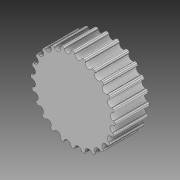
# Autodesk Inventor part: Timing Pulley Generator
Saved by Autodesk Inventor 2022 (Build 260153000, 153)
## iProperties
Created: 2022-01-03
Part Number: Timing Pulley Generator
Material: Generic
Document SubType Name: Modeling
Density: 1 g/cm^3
Appearance: Default
Autodesk Inventor part; units mm, degrees
ref_plane "YZ Plane" through (0, 0, 0) normal (1, 0, 0) x (0, 1, 0)
ref_plane "XZ Plane" through (0, 0, 0) normal (0, 1, 0) x (-1, 0, 0)
ref_plane "XY Plane" through (0, 0, 0) normal (0, 0, 1) x (1, 0, 0)
sketch "Sketch1" plane through (0, 0, 0) normal (0, 0, 1) x (1, 0, 0)
  circle A0 centre (0, 0) radius 11.4592
  dimension "d0" = 22.9183
  constraints: 1 centre point, 1 coincident
  measures "d0" diameter of A0
extrude "Base" add sketch "Sketch1" along normal mid plane 9
sketch "Sketch2" plane through (0, 0, 4.5) normal (0, 0, 1) x (1, 0, 0)
  arc A0 (0.3421, 10.8788) -> (0, 10.8842) centre (0, 0) ccw
  arc A1 (0.7166, 10.2636) -> (0.3421, 10.8788) centre (0.3286, 10.449) ccw
  arc A2 (0.7166, 10.2636) -> (0.8194, 8.8325) centre (2.0255, 9.6384) ccw
  circle A3 centre (0, 0) radius 11.4592 construction
  line L0 (0, 0) -> (0, 10.8842) construction
  line L1 (-3.8998, 12.0715) -> (6.8912, 10.6508) construction
  arc A4 (1.4957, 11.3611) -> (0, 11.4592) centre (0, 0) ccw
  line L2 (0, 10.8842) -> (0, 11.4592)
  line L3 (0, 0) -> (1.4957, 11.3611)
  line L4 (0.8194, 8.8325) -> (1.1525, 8.754)
  dimension "d3" = 0.43
  dimension "d4" = 1.4505
  dimension "d5" = 0.575
  dimension "d6" = 2.6175
  dimension "d13" = 7.5
  dimension "d15" = 0.3422
  dimension "d17" = 0.3422
  dimension "d18" = 84.24
  constraints: 10 end point, 10 point on circle, 4 centre point, 3 tangent, 2 coincident, 2 vertical, 2 vertical alignment, 1 equal length, 1 midpoint, 1 point on line
  measures "d3" radius of A1
  measures "d4" radius of A2
  measures "d5" distance of L0.end L2.end
  measures "d6" distance of L3.end L4.start
  measures "d13" angle of L0 L3
  measures "d17" distance of L4.start L4.end
  measures "d18" angle of L3 L4
extrude "HTD .5 tooth" [suppressed]
mirror "HTD tooth" [suppressed]
pattern_circular "HTD profile" [suppressed]
fillet "HTD fillet" [suppressed]
pattern_circular "HTD teeth" [suppressed]
sketch "Sketch5" plane through (0, 0, 4.5) normal (0, 0, 1) x (1, 0, 0)
  circle A0 centre (0, 0) radius 11.4592 projected
  arc A1 (0.4973, 10.7782) -> (0.1893, 11.0815) centre (0.184, 10.7681) ccw
  arc A2 (0.5093, 10.6307) -> (1.2959, 9.8432) centre (1.4151, 10.7489) ccw
  line L0 (0, 0) -> (0, 11.0832) construction
  line L1 (-3.9984, 12.0844) -> (6.9899, 10.6378) construction
  arc A3 (1.4957, 11.3611) -> (0, 11.4592) centre (0, 0) ccw
  line L2 (0, 11.0832) -> (0, 11.4592)
  line L3 (0, 0) -> (1.4957, 11.3611)
  arc A4 (0.4973, 10.7782) -> (0.5093, 10.6307) centre (2.0165, 10.8274) ccw
  arc A5 (0.1893, 11.0815) -> (0, 11.0832) centre (0, 0) ccw
  arc A6 (2.0981, 11.2654) -> (1.4957, 11.3611) centre (0, 0) ccw construction
  line L4 (2.0165, 10.8274) -> (0, 0) construction
  line L5 (3.5506, 10.8952) -> (3.0796, 9.45) construction
  point P0 (1.4957, 11.3611)
  dimension "d35" = 0.3135
  dimension "d36" = 0.9135
  dimension "d37" = 0.376
  dimension "d39" = 7.5
  dimension "d52" = 1.52
  dimension "d54" = 0.61
  dimension "d61" = 1.531
  dimension "d62" = 1.52
  dimension "d63" = 7.5
  constraints: 13 end point, 12 point on circle, 6 centre point, 4 coincident, 3 point on line, 3 tangent, 2 vertical, 1 equal length, 1 line through centre, 1 midpoint, 6 other
  measures "d35" radius of A1
  measures "d36" radius of A2
  measures "d37" distance of L0.end L2.end
  measures "d39" angle of L0 L3
  measures "d52" radius of A4
  measures "d61" distance of L3.end A2.end
  measures "d62" distance of L5.start L5.end
  measures "d63" angle of L5 L4
extrude "GT2 .5 tooth" cut sketch "Sketch5" against normal through all contours L3 A2 A4 A1 A5 L2 A0 picked at (0.998, 11.1685)
mirror "GT2 tooth" about plane through (0, 0, 0) normal (1, 0, 0) of "GT2 .5 tooth"
pattern_circular "Circular Pattern3" count 24 over 360 about axis through (0, 0, -10) along (0, 0, 1) of "GT2 .5 tooth", "GT2 tooth"
equation "\"d0\" = Pitch_Diameter"
equation "\"d1\" = Width"
equation "\"d3\" = HTD_Root_Fillet_Rad"
equation "\"d6\" = HTD_Belt_Tooth_Height + HTD_Root_to_Pitch_Diameter - HTD_Subtractor"
equation "\"d17\" = d15"
equation "\"d8\" = Width"
equation "\"Pitch\" = 3"
equation "\"Width\" = 9"
equation "\"HTD_Root_Fillet_Rad\" = 0.43"
equation "\"HTD_Tooth_Rad\" = 1.49"
equation "\"HTD_Belt_Height\" = 3.8"
equation "\"HTD_Belt_Tooth_Height\" = 2.06"
equation "\"HTD_Root_to_Pitch_Diameter\" = -0.5 * HTD_Belt_Tooth_Height + 0.5 * HTD_Belt_Height"
equation "\"HTD_Subtractor\" = 0.3125"
equation "\"GT2_Root_Fillet_Rad\" = 0.25"
equation "\"GT2_Root_to_Pitch_Diameter\" = 0.63"
equation "\"GT2_Tooth_Rad\" = 0.85"
equation "\"GT2_Belt_Tooth_Height\" = 1.14"
equation "\"GT2_Belt_Height\" = 2.4"
equation "\"GT2_Middle_Rad\" = 1.52"
equation "\"GT2_Pitch_Offset\" = 0.61"
equation "\"GT2_Teeth_Adjusted\" = 0.04389"
equation "\"Pitch_Diameter\" = 22.918312"
body "Solid1"
